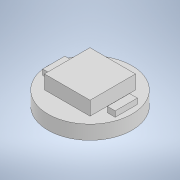
# Autodesk Inventor part: neopixel mini pcb footprint
Saved by Autodesk Inventor 2020 (Build 240168000, 168)
## iProperties
Created: 2020-10-19
Part Number: neopixel mini pcb footprint
Material: Generic
Document SubType Name: Modeling
Designer: mulve
Density: 1 g/cm^3
Appearance: Default
Author: mulve
Autodesk Inventor part; units mm, degrees
ref_plane "YZ Plane" through (0, 0, 0) normal (1, 0, 0) x (0, 1, 0)
ref_plane "XZ Plane" through (0, 0, 0) normal (0, 1, 0) x (-1, 0, 0)
ref_plane "XY Plane" through (0, 0, 0) normal (0, 0, 1) x (1, 0, 0)
sketch "Sketch1" plane through (0, 0, 0) normal (0, 1, 0) x (-1, 0, 0)
  circle A0 centre (0, 0) radius 4.55
  dimension "d0" = 9.1
  constraints: 1 centre point, 1 coincident
  measures "d0" diameter of A0
extrude "Extrusion1" add sketch "Sketch1" along normal blind 1.52
sketch "Sketch2" plane through (0, 1.52, 0) normal (0, 1, 0) x (1, 0, 0)
  line L0 (2.47, -2.465) -> (-2.47, -2.465)
  line L1 (-2.47, -2.465) -> (-2.47, 2.465)
  line L2 (-2.47, 2.465) -> (2.47, 2.465)
  line L3 (2.47, 2.465) -> (2.47, -2.465)
  line L4 (2.47, -2.465) -> (-2.47, 2.465) construction
  line L5 (-2.47, -2.465) -> (2.47, 2.465) construction
  point P0 (0, 0)
  dimension "d3" = 4.94
  dimension "d4" = 4.93
  constraints: 12 end point, 2 midpoint, 2 parallel, 1 horizontal, 1 perpendicular
  measures "d3" distance between parallel lines of L3 L1
  measures "d4" distance of L2.end L0.start
extrude "Extrusion2" add sketch "Sketch2" along normal blind 1.5
sketch "Sketch3" plane through (0, 1.52, 0) normal (0, 1, 0) x (1, 0, 0)
  line L0 (3.935, 1.2) -> (3.085, 1.2)
  line L1 (3.085, 1.2) -> (3.085, -1.2)
  line L2 (3.085, -1.2) -> (3.935, -1.2)
  line L3 (3.935, -1.2) -> (3.935, 1.2)
  line L4 (2.47, -2.465) -> (2.47, 2.465) projected
  circle A0 centre (0, 0) radius 4.55 projected
  line L5 (0, 4.55) -> (0, -4.55) construction
  line L6 (-3.935, 1.2) -> (-3.085, 1.2)
  line L7 (-3.085, 1.2) -> (-3.085, -1.2)
  line L8 (-3.085, -1.2) -> (-3.935, -1.2)
  line L9 (-3.935, -1.2) -> (-3.935, 1.2)
  dimension "d7" = 2.4
  dimension "d8" = 0.85
  dimension "d9" = 0.615
  dimension "d10" = 0.615
  dimension "d11" = 1.2
  dimension "d12" = 1.2
  constraints: 18 end point, 4 symmetric about line, 2 parallel, 2 point on circle, 1 horizontal, 1 perpendicular, 1 vertical
  measures "d7" distance of L2.end L0.start
  measures "d8" distance of L0.start L0.end
  measures "d9" distance between parallel lines of L4 L1
  measures "d10" distance edge to line of A0 L3
  measures "d11" distance from line of A0.centre L0
  measures "d12" distance from line of A0.centre L2
extrude "Extrusion3" add sketch "Sketch3" along normal blind 0.6 contours L3 L2 L1 L0 | L6 L7 L8 L9
equation "\"d9\" = d10"
equation "\"d11\" = d12"
body "Solid1"
